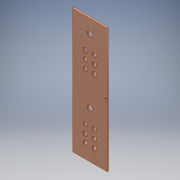
# Autodesk Inventor part: joystick
Saved by Autodesk Inventor 2017 (Build 210142000, 142)
## iProperties
Created: 2017-10-10
Part Number: joystick
Material: Wood (Oak)
Document SubType Name: Modeling
Designer: Felipe
Density: 0.76 g/cm^3
Appearance: White Oak - Natural Medium Gloss
Author: Felipe
Autodesk Inventor part; units mm, degrees
ref_plane "YZ Plane" through (0, 0, 0) normal (1, 0, 0) x (0, 1, 0)
ref_plane "XZ Plane" through (0, 0, 0) normal (0, 1, 0) x (-1, 0, 0)
sketch "Sketch1" plane through (0, 0, 0) normal (0, 1, 0) x (-1, 0, 0)
  line L0 (0, 0) -> (250, 0)
  line L1 (250, 0) -> (250, -900)
  line L2 (250, -900) -> (0, -900)
  line L3 (0, -900) -> (0, 0)
  circle A0 centre (125, -100) radius 20
  circle A1 centre (157.6438, -215) radius 15
  circle A2 centre (157.6438, -275) radius 15
  circle A3 centre (157.6438, -335) radius 15
  circle A4 centre (92.6438, -215) radius 15
  circle A5 centre (92.6438, -275) radius 15
  circle A6 centre (92.6438, -335) radius 15
  line L4 (250, -450) -> (0, -450) construction
  circle A7 centre (157.6438, -680) radius 15
  circle A8 centre (157.6438, -740) radius 15
  circle A9 centre (157.6438, -800) radius 15
  circle A10 centre (92.6438, -680) radius 15
  circle A11 centre (92.6438, -740) radius 15
  circle A12 centre (92.6438, -800) radius 15
  circle A13 centre (125, -565) radius 20
  dimension "d0" = 250
  dimension "d1" = 900
  dimension "d2" = 100
  dimension "d3" = 125
  dimension "d4" = 40
  dimension "d5" = 30
  dimension "d11" = 60
  dimension "d18" = 65
  dimension "d20" = 215
  dimension "d37" = 30
  dimension "d38" = 60
  dimension "d39" = 65
  dimension "d40" = 100
  dimension "d41" = 100
  dimension "d42" = 60
  dimension "d43" = 60
  dimension "d44" = 60
  dimension "d45" = 125
  dimension "d47" = 115
  dimension "d48" = 60
  dimension "d49" = 115
  dimension "d50" = 115
  dimension "d51" = 65
  dimension "d52" = 65
  constraints: 14 centre point, 10 end point, 2 horizontal, 2 midpoint, 2 parallel, 1 equal radius, 1 perpendicular, 1 vertical, 10 other
  measures "d0" distance of L0.start L0.end
  measures "d1" distance of L2.end L0.start
  measures "d2" distance from line of L0 A0.centre
  measures "d3" distance from line of L1 A0.centre
  measures "d4" diameter of A0
  measures "d5" diameter of A1
  measures "d11" distance of A1.centre A2.centre
  measures "d18" distance of A1.centre A4.centre
  measures "d20" distance from line of L0 A1.centre
  measures "d37" diameter of A7
  measures "d38" distance of A7.centre A8.centre
  measures "d39" distance of A7.centre A10.centre
  measures "d40" distance from line of L2 A9.centre
  measures "d41" distance from line of L2 A12.centre
  measures "d42" distance of A2.centre A3.centre
  measures "d43" distance of A8.centre A9.centre
  measures "d44" distance of A11.centre A12.centre
  measures "d45" distance from line of L1 A13.centre
  measures "d47" vertical distance of A10.centre A13.centre
  measures "d48" distance of A11.centre A10.centre
  measures "d49" distance from line of L4 A13.centre
  measures "d50" distance from line of L4 A3.centre
  measures "d51" distance of A9.centre A12.centre
  measures "d52" distance of A8.centre A11.centre
ref_plane "Work Plane1" through (-250, 0, -450) normal (0, 0, 1) x (1, 0, 0)
sketch "Sketch3" plane through (-250, 0, -450) normal (0, 0, 1) x (1, 0, 0)
  circle A0 centre (245, -5) radius 2.5
  circle A1 centre (245, -5) radius 5
  line L0 (250, 0) -> (250, -14.5322) construction
  line L1 (250, 0) -> (0, 0) construction
  dimension "d24" = 5
  dimension "d25" = 10
  constraints: 2 centre point, 2 end point, 2 tangent, 1 coincident, 1 vertical
  measures "d24" diameter of A0
  measures "d25" diameter of A1
extrude "Extrusion2" add sketch "Sketch3" along normal mid plane 15
extrude "Extrusion3" add sketch "Sketch1" along normal blind 10
body "Solid1"
